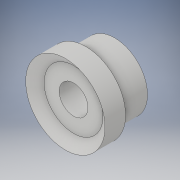
# Autodesk Inventor part: Part4
Saved by Autodesk Inventor 2017 (Build 210142000, 142)
## iProperties
Created: 2017-04-26
Part Number: Part4
Material: Generic
Document SubType Name: Modeling
Designer: 167942
Density: 1 g/cm^3
Appearance: Default
Author: 167942
Autodesk Inventor part; units mm, degrees
ref_plane "YZ Plane" through (0, 0, 0) normal (1, 0, 0) x (0, 1, 0)
ref_plane "XZ Plane" through (0, 0, 0) normal (0, 1, 0) x (-1, 0, 0)
ref_plane "XY Plane" through (0, 0, 0) normal (0, 0, 1) x (1, 0, 0)
sketch "Sketch1" plane through (0, 0, 0) normal (1, 0, 0) x (0, 1, 0)
  line L0 (4.108, 9.9473) -> (-5.9746, 9.9473)
  line L1 (-5.9746, 9.9473) -> (-5.9746, 1.0479)
  line L2 (-5.9746, 1.0479) -> (-7.2571, 1.0479)
  line L3 (-7.2571, 1.0479) -> (-7.2571, -5.9277)
  line L4 (-7.2571, -5.9277) -> (5.4429, -5.9277)
  line L5 (5.4429, -5.9277) -> (5.4429, 5.1848)
  line L6 (5.4429, 5.1848) -> (8.0704, 5.1848)
  line L7 (8.0704, 5.1848) -> (8.0704, 13.1223)
  line L8 (4.108, 9.9473) -> (8.0704, 13.1223)
  point P0 (0, 0)
  dimension "d3" = 19.05
  dimension "d4" = 7.9375
  dimension "d5" = 3.175
  dimension "d6" = 3.9624
  dimension "d7" = 12.7
  constraints: 18 end point, 6 perpendicular, 1 horizontal, 1 vertical
  measures "d3" vertical distance of L4.end L7.end
  measures "d4" distance of L6.end L7.end
  measures "d5" vertical distance of L7.end L0.start
  measures "d6" horizontal distance of L7.end L0.start
  measures "d7" distance between parallel lines of L3 L5
revolve "Revolution1" add sketch "Sketch1" angle 360 about axis through (0, -7.2571, 1.0479) along (0, 0, -1)
sketch "Sketch2" plane through (0, -7.2571, 9.9473) normal (0, 0, 1) x (1, 0, 0)
  circle A0 centre (0, 0) radius 1.2825 projected
  circle A1 centre (0, 0) radius 5.5563
  point P0 (0, 7.2571)
  dimension "d9" = 11.1125
  constraints: 1 centre point, 1 coincident
  measures "d9" diameter of A1
extrude "Extrusion1" cut sketch "Sketch2" against normal blind 7.9375
sketch "Sketch5" plane through (0, -7.2571, 2.0098) normal (0, 0, 1) x (1, 0, 0)
  circle A0 centre (0, 0) radius 3.175
  point P0 (0, 7.2571)
  dimension "d17" = 6.35
  constraints: 1 centre point
  measures "d17" diameter of A0
extrude "Extrusion4" cut sketch "Sketch5" against normal blind 211.1375
body "Solid1"
